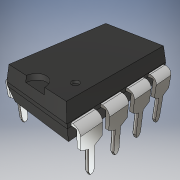
# Autodesk Inventor part: DIL8-Package
Saved by Autodesk Inventor 2018 (Build 220112000, 112)
## iProperties
Created: 2020-04-17
Part Number: DIL8-Package
Material: Všeobecné
Document SubType Name: Modeling
Designer: Jozko Mrkvicka
Density: 1 g/cm^3
Appearance: Výchozí
Author: Jozko Mrkvicka
Autodesk Inventor part; units mm, degrees
ref_plane "YZ Plane" through (0, 0, 0) normal (1, 0, 0) x (0, 1, 0)
ref_plane "XZ Plane" through (0, 0, 0) normal (0, 1, 0) x (-1, 0, 0)
ref_plane "XY Plane" through (0, 0, 0) normal (0, 0, 1) x (1, 0, 0)
sketch "Náčrt1" plane through (0, 0, 0) normal (0, 1, 0) x (-1, 0, 0)
  line L0 (0, 0) -> (6.35, 0)
  line L1 (6.35, 0) -> (6.35, -10.16)
  line L2 (6.35, -10.16) -> (0, -10.16)
  line L3 (0, -10.16) -> (0, 0)
  dimension "d0" = 6.35
  dimension "d1" = 10.16
  constraints: 8 end point, 2 parallel, 1 horizontal, 1 perpendicular
  measures "d0" distance of L1.end L2.end
  measures "d1" distance of L0.end L1.end
extrude "Vysunutí1" add sketch "Náčrt1" along normal blind 3.175
sketch "Náčrt2" plane through (0, 0, 0) normal (1, 0, 0) x (0, 0, -1)
  line L0 (0.3175, 1.7145) -> (2.2225, 1.7145)
  line L1 (2.2225, 1.7145) -> (2.2225, 1.4605)
  line L2 (2.2225, 1.4605) -> (0.3175, 1.4605)
  line L3 (0.3175, 1.4605) -> (0.3175, 1.7145)
  line L4 (0.3175, 1.7145) -> (2.2225, 1.4605) construction
  line L5 (2.2225, 1.7145) -> (0.3175, 1.4605) construction
  line L6 (2.8575, 1.7145) -> (4.7625, 1.7145)
  line L7 (4.7625, 1.7145) -> (4.7625, 1.4605)
  line L8 (4.7625, 1.4605) -> (2.8575, 1.4605)
  line L9 (2.8575, 1.4605) -> (2.8575, 1.7145)
  line L10 (2.8575, 1.7145) -> (4.7625, 1.4605) construction
  line L11 (4.7625, 1.7145) -> (2.8575, 1.4605) construction
  line L12 (5.3975, 1.7145) -> (7.3025, 1.7145)
  line L13 (7.3025, 1.7145) -> (7.3025, 1.4605)
  line L14 (7.3025, 1.4605) -> (5.3975, 1.4605)
  line L15 (5.3975, 1.4605) -> (5.3975, 1.7145)
  line L16 (5.3975, 1.7145) -> (7.3025, 1.4605) construction
  line L17 (7.3025, 1.7145) -> (5.3975, 1.4605) construction
  line L18 (7.9375, 1.7145) -> (9.8425, 1.7145)
  line L19 (9.8425, 1.7145) -> (9.8425, 1.4605)
  line L20 (9.8425, 1.4605) -> (7.9375, 1.4605)
  line L21 (7.9375, 1.4605) -> (7.9375, 1.7145)
  line L22 (7.9375, 1.7145) -> (9.8425, 1.4605) construction
  line L23 (9.8425, 1.7145) -> (7.9375, 1.4605) construction
  point P0 (0, 0)
  point P1 (1.27, 1.5875)
  point P2 (3.81, 1.5875)
  point P3 (6.35, 1.5875)
  point P4 (8.89, 1.5875)
  point P5 (1.27, 1.5875)
  point P6 (3.81, 1.5875)
  point P7 (6.35, 1.5875)
  point P8 (6.35, 1.5875)
  point P9 (8.89, 1.5875)
  point P10 (8.89, 1.5875)
  constraints: 48 end point, 8 midpoint, 8 parallel, 4 horizontal, 4 perpendicular
extrude "Vysunutí2" add sketch "Náčrt2" along normal blind 0.79375
chamfer "Zkosení2" distance 0.254 distance2 1.397 1 edges at (0, 3.175, -5.08) measured on face at (-0.5, 3.175, -5.08)
chamfer "Zkosení3" distance 0.254 distance2 1.397 1 edges at (0, 0, -5.08) measured on face at (-0.5, 0, -5.08)
chamfer "Zkosení4" distance 0.254 distance2 1.397 1 edges at (-6.35, 0, -5.08) measured on face at (-5.85, 0, -5.08)
chamfer "Zkosení5" distance 0.254 distance2 1.397 1 edges at (-6.35, 3.175, -5.08) measured on face at (-5.85, 3.175, -5.08)
chamfer "Zkosení6" distance 0.254 distance2 1.397 1 edges at (-3.175, 3.175, -10.16) measured on face at (-3.175, 3.175, -9.66)
chamfer "Zkosení7" distance 0.254 distance2 1.397 1 edges at (-3.175, 0, -10.16) measured on face at (-3.175, 0, -9.66)
chamfer "Zkosení8" distance 0.254 distance2 1.397 1 edges at (-3.175, 3.175, 0) measured on face at (-3.175, 3.175, -0.5)
chamfer "Zkosení9" distance 0.254 distance2 1.397 1 edges at (-3.175, 0, 0) measured on face at (-3.175, 0, -0.5)
sketch "Náčrt4" plane through (-6.35, 1.778, -10.16) normal (-1, 0, 0) x (0, 0, 1)
  line L0 (0, -0.381) -> (10.16, -0.381) projected
  line L1 (0, -0.381) -> (0, 0) projected
  line L2 (10.16, 0) -> (0, 0) projected
  line L3 (10.16, -0.381) -> (10.16, 0) projected
  line L4 (0, -0.381) -> (10.16, -0.381) projected
  line L5 (0, -0.381) -> (0, 0) projected
  line L6 (10.16, 0) -> (0, 0) projected
  line L7 (10.16, -0.381) -> (10.16, 0) projected
  line L8 (0.3175, -0.0635) -> (0.3175, -0.3175) projected
  line L9 (0.3175, -0.3175) -> (2.2225, -0.3175) projected
  line L10 (2.2225, -0.3175) -> (2.2225, -0.0635) projected
  line L11 (2.2225, -0.0635) -> (0.3175, -0.0635) projected
  line L12 (5.3975, -0.0635) -> (5.3975, -0.3175) projected
  line L13 (5.3975, -0.3175) -> (7.3025, -0.3175) projected
  line L14 (7.3025, -0.3175) -> (7.3025, -0.0635) projected
  line L15 (7.3025, -0.0635) -> (5.3975, -0.0635) projected
  line L16 (7.9375, -0.0635) -> (7.9375, -0.3175) projected
  line L17 (7.9375, -0.3175) -> (9.8425, -0.3175) projected
  line L18 (9.8425, -0.3175) -> (9.8425, -0.0635) projected
  line L19 (9.8425, -0.0635) -> (7.9375, -0.0635) projected
  line L20 (2.8575, -0.0635) -> (2.8575, -0.3175) projected
  line L21 (2.8575, -0.3175) -> (4.7625, -0.3175) projected
  line L22 (4.7625, -0.3175) -> (4.7625, -0.0635) projected
  line L23 (4.7625, -0.0635) -> (2.8575, -0.0635) projected
  line L24 (0, -0.381) -> (10.16, -0.381) projected
  line L25 (0, -0.381) -> (0, 0) projected
  line L26 (10.16, 0) -> (0, 0) projected
  line L27 (10.16, -0.381) -> (10.16, 0) projected
  point P0 (10.16, -1.778)
sketch "Náčrt5" plane through (0, 0, 0) normal (0, -1, 0) x (1, 0, 0)
  circle A0 centre (-5.08, -1.905) radius 0.3175
  point P0 (0, 0)
  dimension "d38" = 0.635
  constraints: 1 centre point, 1 coincident
  measures "d38" diameter of A0
extrude "Vysunutí4" cut sketch "Náčrt5" against normal blind 0.254
sketch "Náčrt6" plane through (0, 0, 0) normal (0, -1, 0) x (1, 0, 0)
  circle A0 centre (-3.175, -0.192418) radius 0.9525
  line L0 (0, -10.16) -> (0, 0)
  dimension "d43" = 1.905
  dimension "d44" = 3.175
  constraints: 2 coincident, 1 centre point
  measures "d43" diameter of A0
  measures "d44" distance from line of point (-3.175, -0.192) L0
extrude "Vysunutí5" cut sketch "Náčrt6" against normal blind 0.508
ref_plane "Pracovní rovina1" through (-6.35, 1.7145, -0.3175) normal (0, 1, 0) x (1, 0, 0)
sketch "Náčrt7" plane through (-6.35, 1.7145, -0.3175) normal (0, 1, 0) x (1, 0, 0)
  line L0 (-0.47625, 0) -> (-0.79375, 0)
  line L1 (-0.79375, 0) -> (-0.79375, 1.905)
  line L2 (-0.79375, 1.905) -> (-0.47625, 1.905)
  line L3 (-0.47625, 1.905) -> (-0.47625, 0)
  line L4 (6.82625, 0) -> (7.14375, 0)
  line L5 (7.14375, 0) -> (7.14375, 1.905)
  line L6 (7.14375, 1.905) -> (6.82625, 1.905)
  line L7 (6.82625, 1.905) -> (6.82625, 0)
  line L8 (-0.47625, 2.54) -> (-0.79375, 2.54)
  line L9 (-0.79375, 2.54) -> (-0.79375, 4.445)
  line L10 (-0.79375, 4.445) -> (-0.47625, 4.445)
  line L11 (-0.47625, 4.445) -> (-0.47625, 2.54)
  line L12 (6.82625, 2.54) -> (7.14375, 2.54)
  line L13 (7.14375, 2.54) -> (7.14375, 4.445)
  line L14 (7.14375, 4.445) -> (6.82625, 4.445)
  line L15 (6.82625, 4.445) -> (6.82625, 2.54)
  line L16 (-0.47625, 5.08) -> (-0.79375, 5.08)
  line L17 (-0.79375, 5.08) -> (-0.79375, 6.985)
  line L18 (-0.79375, 6.985) -> (-0.47625, 6.985)
  line L19 (-0.47625, 6.985) -> (-0.47625, 5.08)
  line L20 (6.82625, 5.08) -> (7.14375, 5.08)
  line L21 (7.14375, 5.08) -> (7.14375, 6.985)
  line L22 (7.14375, 6.985) -> (6.82625, 6.985)
  line L23 (6.82625, 6.985) -> (6.82625, 5.08)
  line L24 (-0.47625, 7.62) -> (-0.79375, 7.62)
  line L25 (-0.79375, 7.62) -> (-0.79375, 9.525)
  line L26 (-0.79375, 9.525) -> (-0.47625, 9.525)
  line L27 (-0.47625, 9.525) -> (-0.47625, 7.62)
  line L28 (6.82625, 7.62) -> (7.14375, 7.62)
  line L29 (7.14375, 7.62) -> (7.14375, 9.525)
  line L30 (7.14375, 9.525) -> (6.82625, 9.525)
  line L31 (6.82625, 9.525) -> (6.82625, 7.62)
  point P0 (6.35, -0.3175)
  point P1 (7.14375, 10.16)
  point P2 (-0.79375, 10.16)
  constraints: 64 end point, 16 parallel, 8 horizontal, 8 perpendicular, 4 coincident
extrude "Vysunutí6" add sketch "Náčrt7" along normal blind 1.905
sketch "Náčrt8" plane through (-6.35, 3.6195, -0.3175) normal (0, 1, 0) x (1, 0, 0)
  line L0 (-0.47625, 1.227463) -> (-0.47625, 0.677537)
  line L1 (-0.79375, 0.677537) -> (-0.79375, 1.227463)
  line L2 (-0.79375, 1.27) -> (-0.47625, 0.635) construction
  line L3 (-0.47625, 1.27) -> (-0.79375, 0.635) construction
  arc A0 (-0.79375, 0.677537) -> (-0.47625, 0.677537) centre (-0.635, 0.9525) ccw
  arc A1 (-0.47625, 1.227463) -> (-0.79375, 1.227463) centre (-0.635, 0.9525) ccw
  line L4 (7.14375, 1.227463) -> (7.14375, 0.677537)
  line L5 (6.82625, 0.677537) -> (6.82625, 1.227463)
  line L6 (6.82625, 1.27) -> (7.14375, 0.635) construction
  line L7 (7.14375, 1.27) -> (6.82625, 0.635) construction
  arc A2 (6.82625, 0.677537) -> (7.14375, 0.677537) centre (6.985, 0.9525) ccw
  arc A3 (7.14375, 1.227463) -> (6.82625, 1.227463) centre (6.985, 0.9525) ccw
  line L8 (-0.47625, 3.767463) -> (-0.47625, 3.217537)
  line L9 (-0.79375, 3.217537) -> (-0.79375, 3.767463)
  line L10 (-0.79375, 3.81) -> (-0.47625, 3.175) construction
  line L11 (-0.47625, 3.81) -> (-0.79375, 3.175) construction
  arc A4 (-0.79375, 3.217537) -> (-0.47625, 3.217537) centre (-0.635, 3.4925) ccw
  arc A5 (-0.47625, 3.767463) -> (-0.79375, 3.767463) centre (-0.635, 3.4925) ccw
  line L12 (7.14375, 3.767463) -> (7.14375, 3.217537)
  line L13 (6.82625, 3.217537) -> (6.82625, 3.767463)
  line L14 (6.82625, 3.81) -> (7.14375, 3.175) construction
  line L15 (7.14375, 3.81) -> (6.82625, 3.175) construction
  arc A6 (6.82625, 3.217537) -> (7.14375, 3.217537) centre (6.985, 3.4925) ccw
  arc A7 (7.14375, 3.767463) -> (6.82625, 3.767463) centre (6.985, 3.4925) ccw
  line L16 (-0.47625, 6.307463) -> (-0.47625, 5.757537)
  line L17 (-0.79375, 5.757537) -> (-0.79375, 6.307463)
  line L18 (-0.79375, 6.35) -> (-0.47625, 5.715) construction
  line L19 (-0.47625, 6.35) -> (-0.79375, 5.715) construction
  arc A8 (-0.79375, 5.757537) -> (-0.47625, 5.757537) centre (-0.635, 6.0325) ccw
  arc A9 (-0.47625, 6.307463) -> (-0.79375, 6.307463) centre (-0.635, 6.0325) ccw
  line L20 (7.14375, 6.307463) -> (7.14375, 5.757537)
  line L21 (6.82625, 5.757537) -> (6.82625, 6.307463)
  line L22 (6.82625, 6.35) -> (7.14375, 5.715) construction
  line L23 (7.14375, 6.35) -> (6.82625, 5.715) construction
  arc A10 (6.82625, 5.757537) -> (7.14375, 5.757537) centre (6.985, 6.0325) ccw
  arc A11 (7.14375, 6.307463) -> (6.82625, 6.307463) centre (6.985, 6.0325) ccw
  line L24 (-0.47625, 8.847463) -> (-0.47625, 8.297537)
  line L25 (-0.79375, 8.297537) -> (-0.79375, 8.847463)
  line L26 (-0.79375, 8.89) -> (-0.47625, 8.255) construction
  line L27 (-0.47625, 8.89) -> (-0.79375, 8.255) construction
  arc A12 (-0.79375, 8.297537) -> (-0.47625, 8.297537) centre (-0.635, 8.5725) ccw
  arc A13 (-0.47625, 8.847463) -> (-0.79375, 8.847463) centre (-0.635, 8.5725) ccw
  line L28 (7.14375, 8.847463) -> (7.14375, 8.297537)
  line L29 (6.82625, 8.297537) -> (6.82625, 8.847463)
  line L30 (6.82625, 8.89) -> (7.14375, 8.255) construction
  line L31 (7.14375, 8.89) -> (6.82625, 8.255) construction
  arc A14 (6.82625, 8.297537) -> (7.14375, 8.297537) centre (6.985, 8.5725) ccw
  arc A15 (7.14375, 8.847463) -> (6.82625, 8.847463) centre (6.985, 8.5725) ccw
  point P0 (6.35, -0.3175)
  point P1 (6.985, 0.9525)
  point P2 (-1.585692, 0.930127)
  point P3 (6.985, 3.4925)
  point P4 (6.985, 3.4925)
  point P5 (6.985, 6.0325)
  point P6 (6.985, 6.0325)
  point P7 (6.985, 8.5725)
  point P8 (6.985, 8.5725)
  point P9 (6.985, 6.0325)
  constraints: 64 end point, 32 point on circle, 27 coincident, 16 centre point, 16 midpoint, 8 parallel
extrude "Vysunutí7" add sketch "Náčrt8" along normal blind 2.54
fillet "Zaoblení1" radius 0.635 4 edges at (0.7937, 1.4605, -1.27) (0.7937, 1.4605, -3.81) (0.7937, 1.4605, -6.35) (0.7937, 1.4605, -8.89)
extrude "Vysunutí8" add sketch "Náčrt4" along normal blind 0.79375 contours L11 L10 L9 L8 | L15 L14 L13 L12 | L19 L18 L17 L16 | L23 L22 L21 L20
fillet "Zaoblení3" radius 0.635 4 edges at (-7.1438, 1.4605, -1.27) (-7.1438, 1.4605, -3.81) (-7.1438, 1.4605, -6.35) (-7.1438, 1.4605, -8.89)
fillet "Zaoblení4" radius 0.3175 4 edges at (0.4762, 1.7145, -1.27) (0.4762, 1.7145, -3.81) (0.4762, 1.7145, -6.35) (0.4762, 1.7145, -8.89)
chamfer "Zkosení105" distance 0.635 angle 30 1 edges at (0.635, 3.6195, -0.3175) measured on face at (0.635, 3.6195, -0.4175)
chamfer "Zkosení106" distance 0.635 angle 30 1 edges at (0.635, 3.6195, -2.2225) measured on face at (0.635, 3.6195, -2.1225)
chamfer "Zkosení107" distance 0.635 angle 30 1 edges at (0.635, 3.6195, -2.8575) measured on face at (0.635, 3.6195, -2.9575)
chamfer "Zkosení108" distance 0.635 angle 30 1 edges at (0.635, 3.6195, -4.7625) measured on face at (0.635, 3.6195, -4.6625)
chamfer "Zkosení109" distance 0.635 angle 30 1 edges at (0.635, 3.6195, -5.3975) measured on face at (0.635, 3.6195, -5.4975)
chamfer "Zkosení110" distance 0.635 angle 30 1 edges at (0.635, 3.6195, -7.3025) measured on face at (0.635, 3.6195, -7.2025)
chamfer "Zkosení111" distance 0.635 angle 30 1 edges at (0.635, 3.6195, -7.9375) measured on face at (0.635, 3.6195, -8.0375)
chamfer "Zkosení112" distance 0.635 angle 30 1 edges at (0.635, 3.6195, -9.8425) measured on face at (0.635, 3.6195, -9.7425)
chamfer "Zkosení121" distance 0.635 angle 30 1 edges at (-6.985, 3.6195, -0.3175) measured on face at (-6.985, 3.6195, -0.4175)
chamfer "Zkosení122" distance 0.635 angle 30 1 edges at (-6.985, 3.6195, -2.2225) measured on face at (-6.985, 3.6195, -2.1225)
chamfer "Zkosení123" distance 0.635 angle 30 1 edges at (-6.985, 3.6195, -2.8575) measured on face at (-6.985, 3.6195, -2.9575)
chamfer "Zkosení124" distance 0.635 angle 30 1 edges at (-6.985, 3.6195, -4.7625) measured on face at (-6.985, 3.6195, -4.6625)
chamfer "Zkosení125" distance 0.635 angle 30 1 edges at (-6.985, 3.6195, -5.3975) measured on face at (-6.985, 3.6195, -5.4975)
chamfer "Zkosení126" distance 0.635 angle 30 1 edges at (-6.985, 3.6195, -7.3025) measured on face at (-6.985, 3.6195, -7.2025)
chamfer "Zkosení127" distance 0.635 angle 30 1 edges at (-6.985, 3.6195, -7.9375) measured on face at (-6.985, 3.6195, -8.0375)
chamfer "Zkosení128" distance 0.635 angle 30 1 edges at (-6.985, 3.6195, -9.8425) measured on face at (-6.985, 3.6195, -9.7425)
chamfer "Zkosení137" distance 0.127 angle 70 2 edges at (-6.985, 6.1595, -0.9525) (-6.985, 6.1595, -1.5875) measured on face at (-6.985, 6.1595, -1.0525) measured on face at (-6.985, 6.1595, -1.4875)
chamfer "Zkosení138" distance 0.127 angle 70 2 edges at (-6.985, 6.1595, -3.4925) (-6.985, 6.1595, -4.1275) measured on face at (-6.985, 6.1595, -3.5925) measured on face at (-6.985, 6.1595, -4.0275)
chamfer "Zkosení139" distance 0.127 angle 70 2 edges at (-6.985, 6.1595, -6.0325) (-6.985, 6.1595, -6.6675) measured on face at (-6.985, 6.1595, -6.5675) measured on face at (-6.985, 6.1595, -6.1325)
chamfer "Zkosení140" distance 0.127 angle 70 2 edges at (-6.985, 6.1595, -8.5725) (-6.985, 6.1595, -9.2075) measured on face at (-6.985, 6.1595, -8.6725) measured on face at (-6.985, 6.1595, -9.1075)
chamfer "Zkosení149" distance 0.127 angle 70 2 edges at (0.635, 6.1595, -9.2075) (0.635, 6.1595, -8.5725) measured on face at (0.635, 6.1595, -8.6725) measured on face at (0.635, 6.1595, -9.1075)
chamfer "Zkosení150" distance 0.127 angle 70 2 edges at (0.635, 6.1595, -6.6675) (0.635, 6.1595, -6.0325) measured on face at (0.635, 6.1595, -6.5675) measured on face at (0.635, 6.1595, -6.1325)
chamfer "Zkosení151" distance 0.127 angle 70 2 edges at (0.635, 6.1595, -4.1275) (0.635, 6.1595, -3.4925) measured on face at (0.635, 6.1595, -3.5925) measured on face at (0.635, 6.1595, -4.0275)
chamfer "Zkosení152" distance 0.127 angle 70 2 edges at (0.635, 6.1595, -1.5875) (0.635, 6.1595, -0.9525) measured on face at (0.635, 6.1595, -1.0525) measured on face at (0.635, 6.1595, -1.4875)
